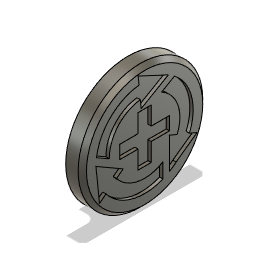
Button Cover Level v3 (Autodesk Fusion 360 design; units mm, degrees)
Autodesk Fusion 360 part; units mm, degrees
sketch "Sketch1" plane through (0, 0, 0) normal (1, 0, 0) x (0, 0, -1)
  circle A0 centre (0, 0) radius 4
  line L0 (2, 2) -> (-2, 2)
  line L1 (-2, 2) -> (-2, -2)
  line L2 (-2, -2) -> (2, -2)
  line L3 (2, -2) -> (2, 2)
  line L4 (2, 2) -> (-2, -2) construction
  line L5 (-2, 2) -> (2, -2) construction
  dimension "d1" = 8
  dimension "d2" = 4
  dimension "d3" = 4
  constraint coincident A0.centre origin
  constraint horizontal L0
  constraint perpendicular L0 L1
  constraint parallel L0 L2
  constraint parallel L1 L3
  constraint coincident L4 A0.centre
  constraint coincident L5 A0.centre
  measures "d1" diameter of A0
  measures "d2" distance of L0.start L0.end
  measures "d3" distance of L0.start L2.end
extrude "Extrude1" add sketch "Sketch1" along normal blind 2
sketch "Sketch2" plane through (2, 0, 0) normal (1, 0, 0) x (0, 0, -1)
  line L0 (2, 2) -> (2, -2)
  line L1 (2, -2) -> (-2, -2)
  line L2 (-2, -2) -> (-2, 2)
  line L3 (-2, 2) -> (2, 2)
  circle A0 centre (0, 0) radius 4
  circle A1 centre (0, 0) radius 7.5
  dimension "d6" = 15
  constraint coincident A0.centre A1.centre
  measures "d6" diameter of A1
extrude "Extrude2" add sketch "Sketch2" along normal blind 2 contours L0 L1 L2 L3 | A0 | A1
fillet "Fillet1" radius 1 1 edges at (2, -1.4465, 3.7293)
chamfer "Chamfer1" distance 0.5 angle 45 1 edges at (4, -2.7121, 6.9925)
sketch "Sketch3" plane through (4, 0, 0) normal (1, 0, 0) x (0, 0, -1)
  circle A0 centre (0, 0) radius 7
  circle A1 centre (0, 0) radius 5.85
  circle A2 centre (0, 0) radius 4.25
  line L0 (0.8, 3) -> (-0.8, 3)
  line L1 (-0.8, 3) -> (-0.8, -3)
  line L2 (-0.8, -3) -> (0.8, -3)
  line L3 (0.8, -3) -> (0.8, 3)
  line L4 (0.8, 3) -> (-0.8, -3) construction
  line L5 (-0.8, 3) -> (0.8, -3) construction
  line L6 (3, -0.8) -> (-3, -0.8)
  line L7 (-3, -0.8) -> (-3, 0.8)
  line L8 (-3, 0.8) -> (3, 0.8)
  line L9 (3, 0.8) -> (3, -0.8)
  line L10 (3, -0.8) -> (-3, 0.8) construction
  line L11 (-3, -0.8) -> (3, 0.8) construction
  circle A3 centre (0, 0) radius 3 construction
  line L12 (-1.5, 2.5981) -> (2.8494, 5.1092)
  line L13 (3, 0) -> (3, -5.0222)
  line L14 (-1.5, -2.5981) -> (-5.8494, -0.087)
  line L15 (-5.8494, -0.087) -> (-5.4432, -4.1586)
  line L16 (-5.4432, -4.1586) -> (-2.5825, -1.9731)
  line L17 (2.8494, 5.1092) -> (-0.7748, 6.8053)
  line L18 (-0.7748, 6.8053) -> (-0.4175, 3.2231)
  line L19 (6.3231, -2.6346) -> (3, -1.25)
  line L20 (-2.5825, -1.9731) -> (0, 0) construction
  line L21 (3, -1.25) -> (0, 0) construction
  line L22 (-0.4175, 3.2231) -> (0, 0) construction
  line L23 (3, -5.0222) -> (6.3231, -2.6346)
  circle A4 centre (0, 0) radius 3.25 construction
  line L24 (2.0491, 3.7234) -> (3.5943, 4.6155)
  line L25 (2.2, -3.6363) -> (2.2, -5.4206)
  line L26 (-5.7943, 0.805) -> (-4.2491, -0.0871)
  dimension "d12" = 1.6
  dimension "d13" = 1.6
  dimension "d14" = 6
  dimension "d15" = 6
  dimension "d16" = 1.6
  dimension "d17" = 120
  dimension "d18" = 120
  dimension "d20" = 3.6
  dimension "d21" = 3.6
  dimension "d22" = 8.5
  dimension "d23" = 6
  dimension "d24" = 1
  dimension "d25" = 0.8
  dimension "d26" = 0.8
  dimension "d27" = 0.8
  dimension "d30" = 3.6
  constraint concentric A0 A1
  constraint concentric A1 A2
  constraint horizontal L0
  constraint perpendicular L0 L1
  constraint parallel L0 L2
  constraint parallel L1 L3
  constraint coincident L4 A0.centre
  constraint coincident L5 A0.centre
  constraint coincident A0.centre A1.centre
  constraint horizontal L6
  constraint perpendicular L6 L7
  constraint parallel L6 L8
  constraint parallel L7 L9
  constraint coincident L10 A0.centre
  constraint coincident L11 A0.centre
  constraint concentric A2 A3
  constraint vertical L13
  constraint tangent A3 L14
  constraint tangent A3 L12
  constraint tangent A3 L13
  constraint coincident A1 L13.end
  constraint coincident A1 L12.end
  constraint coincident A1 L14.end
  constraint coincident A3 L13.start
  constraint coincident A3 L14.start
  constraint coincident A3 L12.start
  constraint coincident L14 L16.end
  constraint coincident L12 L18.end
  constraint parallel L15 L18
  constraint coincident L13 L19.end
  constraint collinear L19 L21
  constraint collinear L16 L20
  constraint coincident L19.end A4
  constraint coincident L16.end A4
  constraint coincident L18.end A4
  constraint coincident A2 L24.start
  constraint coincident A1 L24.end
  constraint coincident A2 L25.start
  constraint coincident A1 L25.end
  constraint parallel L13 L25
  constraint coincident A1 L26.start
  constraint coincident A2 L26.end
  constraint parallel L14 L26
  constraint parallel L12 L24
  measures "d12" distance of L0.start L0.end
  measures "d13" distance of L6.start L8.end
  measures "d14" distance of L7.end L8.end
  measures "d15" distance of L0.start L2.end
  measures "d16" distance of A1 A2
  measures "d17" angle of L12 L13
  measures "d18" angle of L12 L14
  measures "d20" distance of L19.start L19.end
  measures "d21" distance of L17.end L18.end
  measures "d22" diameter of A2
  measures "d23" diameter of A3
  measures "d24" distance of A2 A4
  measures "d25" distance of L12 L24
  measures "d26" distance of L13 L25
  measures "d27" distance of L14 L26
  measures "d30" distance of L15.end L16.end
extrude "Extrude3" cut sketch "Sketch3" against normal blind 0.4 contours A1 A2 L19 L24 | A1 L19 L23 | A1 A2 L13 L19 L23 | A1 L17 | A1 A2 L12 L17 L18 | A1 L23 | A2 L13 L19 | A1 L17 L18 | A2 L12 L18 | A1 A2 L18 L26 | A1 A2 L16 L25 | L3 L6 L8 L9 L13 | L0 L1 L3 L8 | A1 L15 L16 | A1 A2 L14 L15 L16 | A2 L14 L16 | L1 L3 L6 L8 | L1 L2 L3 L6 | A1 L15 | L1 L6 L7 L8
